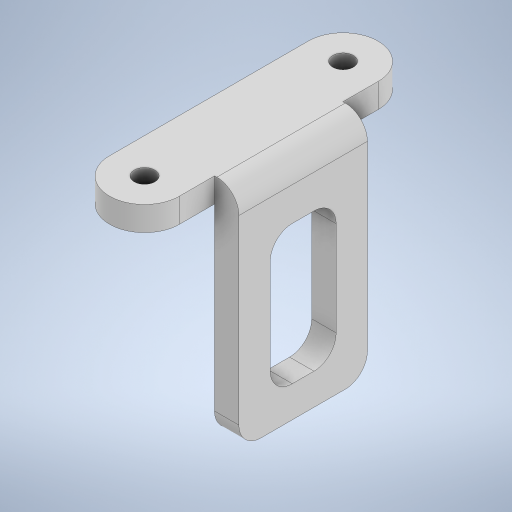
# Autodesk Inventor part: frontbackmount
Saved by Autodesk Inventor 2023 (Build 270158000, 158)
## iProperties
Created: 2022-12-04
Part Number: frontbackmount
Material: Generic
Document SubType Name: Modeling
Designer: user
Density: 1 g/cm^3
Appearance: Default
Author: user
Autodesk Inventor part; units mm, degrees
ref_plane "YZ Plane" through (0, 0, 0) normal (1, 0, 0) x (0, 1, 0)
ref_plane "XZ Plane" through (0, 0, 0) normal (0, 1, 0) x (-1, 0, 0)
ref_plane "XY Plane" through (0, 0, 0) normal (0, 0, 1) x (1, 0, 0)
sketch "Sketch1" plane through (0, 0, 0) normal (0, 1, 0) x (-1, 0, 0)
  circle A0 centre (0, 0) radius 1.4732
  circle A1 centre (0, -28.4988) radius 1.4732
  circle A2 centre (0, 0) radius 5.0165
  circle A3 centre (0, -28.4988) radius 5.0165
  line L0 (5.0165, 0) -> (5.0165, -28.4988)
  line L1 (-5.0165, 0) -> (-5.0165, -28.4988)
  dimension "d0" = 2.9464
  dimension "d2" = 2.9464
  dimension "d3" = 10.033
  dimension "d4" = 10.033
  constraints: 4 centre point, 4 end point, 4 point on circle, 3 coincident, 2 tangent
  measures "d0" diameter of A0
  measures "d2" diameter of A1
  measures "d3" diameter of A2
  measures "d4" diameter of A3
extrude "Extrusion1" add sketch "Sketch1" along normal blind 3.5
sketch "Sketch2" plane through (5.0165, 0, 0) normal (1, 0, 0) x (0, 0, -1)
  line L0 (0, 0) -> (28.4988, 0) projected
  line L1 (0, 0) -> (5.0292, 0)
  line L2 (28.4988, 0) -> (28.4988, 3.5) projected
  line L3 (28.4988, 0) -> (23.4696, 0)
  line L4 (23.4696, 0) -> (5.0292, 0)
  line L5 (5.0292, 0) -> (5.0292, -25.7302)
  line L6 (8.2042, -28.9052) -> (20.2946, -28.9052)
  line L7 (23.4696, -25.7302) -> (23.4696, 0)
  line L8 (5.0292, 0) -> (23.4696, 0)
  line L9 (5.0292, 0) -> (11.3792, 0)
  line L10 (23.4696, 0) -> (17.1196, 0)
  line L11 (5.0292, -28.9052) -> (11.3792, -28.9052)
  arc A0 (5.0292, -25.7302) -> (8.2042, -28.9052) centre (8.2042, -25.7302) ccw
  arc A1 (20.2946, -28.9052) -> (23.4696, -25.7302) centre (20.2946, -25.7302) ccw
  line L12 (15.8041, -24.4147) -> (12.694, -24.4147)
  line L13 (12.694, -4.4898) -> (15.8041, -4.4898)
  line L14 (18.9791, -7.6648) -> (18.9791, -21.2397)
  line L15 (9.519, -21.2397) -> (9.519, -7.6648)
  arc A2 (12.694, -4.4898) -> (9.519, -7.6648) centre (12.694, -7.6648) ccw
  arc A3 (9.519, -21.2397) -> (12.694, -24.4147) centre (12.694, -21.2397) ccw
  arc A4 (15.8041, -24.4147) -> (18.9791, -21.2397) centre (15.8041, -21.2397) ccw
  arc A5 (18.9791, -7.6648) -> (15.8041, -4.4898) centre (15.8041, -7.6648) ccw
  point P0 (9.519, -24.4147)
  dimension "d7" = 5.0292
  dimension "d8" = 5.0292
  dimension "d9" = 28.9052
  dimension "d10" = 6.35
  dimension "d14" = 6.35
  dimension "d17" = 3.175
  dimension "d23" = 6.35
  dimension "d25" = 3.175
  constraints: 28 end point, 12 point on circle, 12 tangent, 9 point on line, 6 centre point, 4 equal radius, 3 perpendicular, 2 parallel, 1 collinear, 1 horizontal, 1 vertical
  measures "d7" distance of L0.start L1.end
  measures "d8" distance of L0.end L3.end
  measures "d9" distance of L1.end L11.start
  measures "d10" distance of L1.end L9.end
  measures "d14" distance of L11.start L11.end
  measures "d17" radius of A0
  measures "d23" distance of L11.start point (9.519, -24.415)
  measures "d25" radius of A2
extrude "Extrusion4" add sketch "Sketch2" along normal blind 3.5
sketch "Sketch4" plane through (5.0165, 0, -5.0292) normal (0, 1, 0) x (1, 0, 0)
  line L0 (0, 0) -> (3.5, 0) projected
  line L1 (3.5, 15.2654) -> (3.5, 18.4404) projected
  line L2 (3.5, 0) -> (3.5, 18.4404)
  line L3 (0, 18.4404) -> (3.5, 18.4404) projected
  line L4 (3.5, 18.4404) -> (0, 18.4404)
  line L5 (0, 18.4404) -> (0, 0)
  line L6 (0, 0) -> (3.5, 0)
  point P0 (-5.0165, -5.0292)
  constraints: 8 end point, 3 perpendicular, 1 collinear
extrude "Extrusion5" add sketch "Sketch4" along normal blind 3.5
fillet "Fillet3" radius 3.175 1 edges at (8.5165, 3.5, -14.2494)
body "Solid1"
